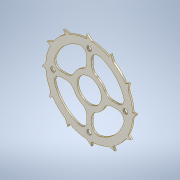
# Autodesk Inventor part: Wood Magnets  (UNI) V1.0.
Saved by Autodesk Inventor 2022.1 (Build 261234020, 234B)
## iProperties
Created: 2022-03-16
Part Number: Wood Magnets  (UNI) V1.0.
Material: Titanium
Document SubType Name: Modeling
Designer: NCai2
Density: 4.51 g/cm^3
Appearance: Titanium
Mass: 5.57938 g
Surface Area: 30.6065 cm^2
Volume: 1.23711 cm^3
Author: NCai2
Autodesk Inventor part; units mm, degrees
ref_plane "YZ Plane" through (0, 0, 0) normal (1, 0, 0) x (0, 1, 0)
ref_plane "XZ Plane" through (0, 0, 0) normal (0, 1, 0) x (-1, 0, 0)
ref_plane "XY Plane" through (0, 0, 0) normal (0, 0, 1) x (1, 0, 0)
sketch "Sketch1" plane through (0, 0, 0) normal (0, 0, 1) x (1, 0, 0)
  circle A0 centre (0, 0) radius 28.575
  circle A1 centre (0, 0) radius 23.8125 construction
  circle A2 centre (0, 0) radius 11.1125
  line L0 (0, 0) -> (0, 28.575) construction
  circle A3 centre (0, 23.8125) radius 1.5
  line L1 (-1.5875, 10.9985) -> (-1.5875, 28.5309)
  line L2 (1.5875, 10.9985) -> (1.5875, 28.5309)
  arc A4 (7.1541, 22.7124) -> (1.5875, 18.6296) centre (5.868, 18.6296) ccw
  arc A5 (-1.5875, 18.6296) -> (-7.1541, 22.7124) centre (-5.868, 18.6296) ccw
  arc A6 (1.5875, 15.1594) -> (4.8218, 10.0119) centre (7.3009, 15.1594) ccw
  arc A7 (-4.8218, 10.0119) -> (-1.5875, 15.1594) centre (-7.3009, 15.1594) ccw
  arc A8 (-15.1594, 1.5875) -> (-10.0119, 4.8218) centre (-15.1594, 7.3009) ccw
  line L3 (-10.9985, 1.5875) -> (-28.5309, 1.5875)
  line L4 (-10.9985, -1.5875) -> (-28.5309, -1.5875)
  arc A9 (-10.0119, -4.8218) -> (-15.1594, -1.5875) centre (-15.1594, -7.3009) ccw
  arc A10 (-22.7124, 7.1541) -> (-18.6296, 1.5875) centre (-18.6296, 5.868) ccw
  arc A11 (-18.6296, -1.5875) -> (-22.7124, -7.1541) centre (-18.6296, -5.868) ccw
  circle A12 centre (-23.8125, 0) radius 1.5
  arc A13 (-1.5875, -15.1594) -> (-4.8218, -10.0119) centre (-7.3009, -15.1594) ccw
  line L5 (-1.5875, -10.9985) -> (-1.5875, -28.5309)
  line L6 (1.5875, -10.9985) -> (1.5875, -28.5309)
  arc A14 (4.8218, -10.0119) -> (1.5875, -15.1594) centre (7.3009, -15.1594) ccw
  arc A15 (-7.1541, -22.7124) -> (-1.5875, -18.6296) centre (-5.868, -18.6296) ccw
  arc A16 (1.5875, -18.6296) -> (7.1541, -22.7124) centre (5.868, -18.6296) ccw
  circle A17 centre (0, -23.8125) radius 1.5
  arc A18 (15.1594, -1.5875) -> (10.0119, -4.8218) centre (15.1594, -7.3009) ccw
  line L7 (10.9985, -1.5875) -> (28.5309, -1.5875)
  line L8 (10.9985, 1.5875) -> (28.5309, 1.5875)
  arc A19 (10.0119, 4.8218) -> (15.1594, 1.5875) centre (15.1594, 7.3009) ccw
  arc A20 (22.7124, -7.1541) -> (18.6296, -1.5875) centre (18.6296, -5.868) ccw
  arc A21 (18.6296, 1.5875) -> (22.7124, 7.1541) centre (18.6296, 5.868) ccw
  circle A22 centre (23.8125, 0) radius 1.5
  circle A23 centre (0, 0) radius 7.9375
  arc A24 (-7.1541, 22.7124) -> (-22.7124, 7.1541) centre (0, 0) ccw
  arc A25 (-23.2466, 5.1606) -> (-17.5518, -16.0925) centre (0, 0) ccw
  arc A26 (-16.0925, -17.5518) -> (5.1606, -23.2466) centre (0, 0) ccw
  arc A27 (7.1541, -22.7124) -> (22.7124, -7.1541) centre (0, 0) ccw
  arc A28 (23.2466, -5.1606) -> (17.5518, 16.0925) centre (0, 0) ccw
  arc A29 (16.0925, 17.5518) -> (-5.1606, 23.2466) centre (0, 0) ccw
  line L9 (-1.5875, 28.5309) -> (-1.5875, 31.0709)
  line L10 (-1.5875, 31.0709) -> (1.5875, 28.5309)
  line L11 (-16.9102, 26.1144) -> (-12.8906, 25.5022)
  line L12 (-15.6402, 23.9147) -> (-16.9102, 26.1144)
  line L13 (-27.7019, 14.1606) -> (-23.9147, 15.6402)
  line L14 (-25.5022, 12.8906) -> (-27.7019, 14.1606)
  line L15 (-31.0709, -1.5875) -> (-28.5309, 1.5875)
  line L16 (-28.5309, -1.5875) -> (-31.0709, -1.5875)
  line L17 (-26.1144, -16.9102) -> (-25.5022, -12.8906)
  line L18 (-23.9147, -15.6402) -> (-26.1144, -16.9102)
  line L19 (-14.1606, -27.7019) -> (-15.6402, -23.9147)
  line L20 (-12.8906, -25.5022) -> (-14.1606, -27.7019)
  line L21 (1.5875, -31.0709) -> (-1.5875, -28.5309)
  line L22 (1.5875, -28.5309) -> (1.5875, -31.0709)
  line L23 (16.9102, -26.1144) -> (12.8906, -25.5022)
  line L24 (15.6402, -23.9147) -> (16.9102, -26.1144)
  line L25 (27.7019, -14.1606) -> (23.9147, -15.6402)
  line L26 (25.5022, -12.8906) -> (27.7019, -14.1606)
  line L27 (31.0709, 1.5875) -> (28.5309, -1.5875)
  line L28 (28.5309, 1.5875) -> (31.0709, 1.5875)
  line L29 (26.1144, 16.9102) -> (25.5022, 12.8906)
  line L30 (23.9147, 15.6402) -> (26.1144, 16.9102)
  line L31 (14.1606, 27.7019) -> (15.6402, 23.9147)
  line L32 (12.8906, 25.5022) -> (14.1606, 27.7019)
  arc A30 (-22.7124, -7.1541) -> (-7.1541, -22.7124) centre (0, 0) ccw
  arc A31 (7.1541, -22.7124) -> (22.7124, -7.1541) centre (0, 0) ccw
  arc A32 (23.0011, 6.1631) -> (7.1541, 22.7124) centre (0, 0) ccw
  arc A33 (-7.1541, 22.7124) -> (-22.7124, 7.1541) centre (0, 0) ccw
  point P0 (-1.5875, 15.1594)
  point P1 (-4.8218, 10.0119)
  point P2 (-10.0119, 4.8218)
  point P3 (-1.5875, 18.6296)
  point P4 (1.5875, -15.1594)
  point P5 (4.8218, -10.0119)
  point P6 (10.0119, -4.8218)
  point P7 (-7.072, -22.7381)
  point P8 (-16.1558, -17.4936)
  point P9 (1.5875, -18.6296)
  point P10 (-28.5309, 1.5875)
  point P11 (-23.9147, -15.6402)
  point P12 (-1.5875, -28.5309)
  point P13 (1.5875, -28.5309)
  point P14 (23.9147, -15.6402)
  point P15 (25.5022, -12.8906)
  point P16 (25.5022, 12.8906)
  point P17 (23.9147, 15.6402)
  point P18 (15.1594, 1.5875)
  point P19 (7.072, -22.7381)
  point P20 (18.6296, 1.5875)
  point P21 (-15.1594, -1.5875)
  point P22 (-10.0119, -4.8218)
  point P23 (-4.8218, -10.0119)
  point P24 (-23.2278, -5.2445)
  point P25 (-22.7124, -7.1541)
  point P26 (-18.6296, -1.5875)
  point P27 (7.1541, 22.7124)
  point P28 (-23.7595, -1.5875)
  point P29 (16.0925, 17.5518)
  point P30 (17.5518, 16.0925)
  point P31 (22.7124, 7.1541)
  point P32 (-7.1541, -22.7124)
  point P33 (-16.0925, -17.5518)
  point P34 (-17.5518, -16.0925)
  point P35 (22.7124, -7.1541)
  point P36 (7.1541, -22.7124)
  dimension "d0" = 57.15
  dimension "d1" = 47.625
  dimension "d2" = 22.225
  dimension "d3" = 3
  dimension "d4" = 1.5875
  dimension "d5" = 1.5875
  dimension "d8" = 360
  dimension "d10" = 15.875
  dimension "d13" = 360
  dimension "d15" = 2.54
  dimension "d18" = 360
  constraints: 66 end point, 60 point on circle, 33 centre point, 9 point on line, 6 symmetric about line, 6 tangent, 5 concentric, 4 coincident, 2 parallel, 2 vertical, 190 other
  measures "d1" diameter of A1
  measures "d2" diameter of A2
  measures "d3" diameter of A3
  measures "d4" distance between parallel lines of L0 L1
  measures "d5" distance between parallel lines of L0 L2
  measures "d10" diameter of A23
  measures "d15" distance of L1.end L9.end
extrude "Extrusion1" add sketch "Sketch1" along normal blind 1 contours A0 L7 A28 A22 L8 | A0 L28 L27 | L8 A28 A32 A29 L2 A0 | A0 L6 A16 A27 A20 L7 | A0 L30 L29 | A28 A22 L7 A2 L8 | L8 A21 A28 | L26 L25 A0 | A0 L32 L31 | L8 A2 A19 | L24 L23 A0 | A18 A2 L7 | A2 | L2 A29 A3 L1 A0 | A0 L9 L10 | A2 L2 A6 | L22 L21 A0 | A0 L5 A26 A17 L6 | A14 L6 A2 | L6 A26 A17 L5 A2 | L1 A5 A24 A10 L3 A0 | A29 A4 L2 | L2 A2 L1 A29 A3 | A0 L4 A25 A30 A26 L5 | A0 L12 L11 | A2 A7 L1 | L20 L19 A0 | A26 A15 L5 | L5 A13 A2 | A0 L14 L13 | A2 L3 A8 | L18 L17 A0 | A9 L4 A2 | A2 L4 A25 A12 L3 | L3 A25 A12 L4 A0 | A0 L16 L15 | A25 L4 A11
body "Solid1"
